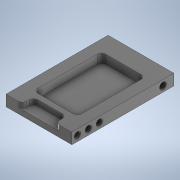
# Autodesk Inventor part: Cockpit_lower_back_door
Saved by Autodesk Inventor 2020 (Build 240168000, 168)
## iProperties
Created: 2021-06-08
Part Number: Cockpit_lower_back_door
Material: アセタール樹脂、黒
Document SubType Name: Modeling
Designer: Masato Kubotera
Density: 1.425 g/cm^3
Appearance: 滑らか - 黒
Description: POM T5
Author: Masato Kubotera
Title: Cockpit_vertical_frame_07
Autodesk Inventor part; units mm, degrees
ref_plane "YZ Plane" through (0, 0, 0) normal (1, 0, 0) x (0, 1, 0)
ref_plane "XZ Plane" through (0, 0, 0) normal (0, 1, 0) x (-1, 0, 0)
ref_plane "XY Plane" through (0, 0, 0) normal (0, 0, 1) x (1, 0, 0)
sketch "スケッチ1" plane through (0, 0, 0) normal (0, 0, 1) x (1, 0, 0)
  line L0 (0, 46.5) -> (30, 46.5)
  line L1 (0, 0) -> (30, 0)
  line L2 (0, 0) -> (0, 46.5)
  line L3 (30, 0) -> (30, 46.5)
  line L4 (7.5, 0) -> (7.5, 5)
  line L5 (7.5, 5) -> (22.5, 5)
  line L6 (15, 0) -> (15, 46.5) construction
  line L7 (22.5, 0) -> (22.5, 5)
  line L8 (5, 38.5) -> (25, 38.5)
  line L9 (25, 38.5) -> (25, 7.5)
  line L10 (25, 7.5) -> (5, 7.5)
  line L11 (5, 38.5) -> (5, 7.5)
  point P0 (22.5, 0)
  dimension "d2" = 30
  dimension "d38" = 46.5
  dimension "d61" = 15
  dimension "d62" = 5
  dimension "d66" = 5
  dimension "d67" = 8
  dimension "d68" = 2.5
  constraints: 24 end point, 4 perpendicular, 4 symmetric about line, 2 midpoint, 2 parallel, 2 vertical, 1 coincident, 1 horizontal, 1 point on line
  measures "d2" distance of L0.start L0.end
  measures "d38" distance of L1.start L0.start
  measures "d61" distance of L4.end L5.end
  measures "d62" distance of L7.start L5.end
  measures "d66" distance between parallel lines of L2 L11
  measures "d67" distance between parallel lines of L8 L0
  measures "d68" distance between parallel lines of L10 L5
extrude "押し出し1" add sketch "スケッチ1" along normal blind 5 contours L0 L3 L1 L7 L5 L4 L2
sketch "スケッチ4" plane through (30, 0, 0) normal (1, 0, 0) x (0, 0, -1)
  line L0 (0, 46.5) -> (-5, 46.5) projected
  line L1 (-2.5, 46.5) -> (-2.5, 0) construction
  line L2 (0, 0) -> (-5, 0) projected
  point P0 (0, 0)
  point P1 (-2.5, 41.5)
  point P2 (-2.5, 2.5)
  point P3 (-2.5, 7.5)
  point P4 (-2.5, 12.5)
  dimension "d22" = 5
  dimension "d40" = 2.5
  dimension "d41" = 5
  dimension "d42" = 5
  dimension "d60" = 29
  constraints: 4 point on line, 2 end point, 2 midpoint
  measures "d22" distance of L1.start point (-2.5, 41.5)
  measures "d40" distance of L1.end point (-2.5, 2.5)
  measures "d41" distance of point (-2.5, 2.5) point (-2.5, 7.5)
  measures "d42" distance of point (-2.5, 7.5) point (-2.5, 12.5)
  measures "d60" distance of point (-2.5, 12.5) point (-2.5, 41.5)
hole "穴1" at (30, 41.5, 2.5) direction (-1, 0, 0) diameter 3.1 depth 3
sketch "スケッチ5" plane through (0, 0, 0) normal (-1, 0, 0) x (0, 0, 1)
  circle A0 centre (2.5, 41.5) radius 1.55 projected
  line L0 (0, 0) -> (5, 0) projected
  line L1 (2.5, 0) -> (2.5, 46.5) construction
  line L2 (0, 46.5) -> (5, 46.5) projected
  point P0 (2.5, 2.5)
  point P1 (2.5, 7.5)
  point P2 (2.5, 12.5)
  point P3 (4.05, 32)
  point P4 (0.95, 32)
  dimension "d50" = 2.5
  dimension "d51" = 5
  dimension "d52" = 5
  constraints: 3 point on line, 2 end point, 2 midpoint, 1 coincident, 1 other
  measures "d50" distance of point (2.5, 2.5) L1.start
  measures "d51" distance of point (2.5, 7.5) point (2.5, 2.5)
  measures "d52" distance of point (2.5, 12.5) point (2.5, 7.5)
hole "穴2" at (0, 41.5, 2.5) direction (1, 0, 0) diameter 3.1 depth 3
hole "穴5" at (30, 2.5, 2.5) at (30, 12.5, 2.5) at (30, 7.5, 2.5) direction (-1, 0, 0) diameter 2.9 depth 3
hole "穴6" at (0, 2.5, 2.5) at (0, 7.5, 2.5) at (0, 12.5, 2.5) direction (1, 0, 0) diameter 2.9 depth 3
extrude "押し出し2" add sketch "スケッチ1" along normal blind 2.5 contours L4 L5 L7 L1
fillet "フィレット3" radius 2 8 edges at (7.5, 5, 3.75) (7.5, 0, 3.75) (22.5, 5, 3.75) (22.5, 0, 3.75) (5, 38.5, 2.5) (25, 38.5, 2.5) (5, 7.5, 2.5) (25, 7.5, 2.5)
extrude "押し出し3" add sketch "スケッチ1" along normal blind 1 contours L8 L9 L10 L11
equation "\"d41\" = d42"
equation "\"d50\" = d40"
equation "\"d51\" = d41"
equation "\"d52\" = d42"
